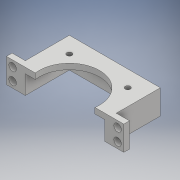
# Autodesk Inventor part: Step motor mount Top
Saved by Autodesk Inventor 2018 (Build 220112000, 112)
## iProperties
Created: 2019-03-21
Part Number: Step motor mount Top
Material: Типовые
Document SubType Name: Modeling
Designer: cosko
Density: 1 g/cm^3
Appearance: По умолчанию
Author: cosko
Autodesk Inventor part; units mm, degrees
ref_plane "YZ Plane" through (0, 0, 0) normal (1, 0, 0) x (0, 1, 0)
ref_plane "XZ Plane" through (0, 0, 0) normal (0, 1, 0) x (-1, 0, 0)
ref_plane "XY Plane" through (0, 0, 0) normal (0, 0, 1) x (1, 0, 0)
sketch "Эскиз1" plane through (0, 0, 0) normal (0, 0, 1) x (1, 0, 0)
  line L0 (-21.15, -21.15) -> (21.15, -21.15)
  line L1 (21.15, -21.15) -> (21.15, 21.15)
  line L2 (21.15, 21.15) -> (-21.15, 21.15)
  line L3 (-21.15, 21.15) -> (-21.15, -21.15)
  line L4 (-21.15, -21.15) -> (21.15, 21.15) construction
  line L5 (21.15, -21.15) -> (-21.15, 21.15) construction
  line L6 (0, 21.15) -> (15.5, 21.15) construction
  line L7 (15.5, 21.15) -> (-15.5, 21.15) construction
  line L8 (21.15, 0) -> (21.15, -15.5) construction
  line L9 (21.15, -15.5) -> (21.15, 15.5) construction
  line L10 (15.5, 21.15) -> (15.5, -21.15) construction
  line L11 (21.15, -15.5) -> (-21.15, -15.5) construction
  line L12 (21.15, 15.5) -> (-21.15, 15.5) construction
  line L13 (-15.5, 21.15) -> (-15.5, -21.15) construction
  circle A0 centre (-15.5, 15.5) radius 1.35
  circle A1 centre (-15.5, -15.5) radius 1.35
  circle A2 centre (15.5, -15.5) radius 1.35
  circle A3 centre (15.5, 15.5) radius 1.35
  circle A4 centre (0, 0) radius 11
  circle A5 centre (0, 0) radius 2.5
  circle A6 centre (0, 0) radius 2.25
  dimension "d0" = 42.3
  dimension "d1" = 42.3
  dimension "d3" = 31
  dimension "d4" = 15.5
  dimension "d5" = 31
  dimension "d6" = 2.7
  dimension "d7" = 2.7
  dimension "d8" = 2.7
  dimension "d9" = 2.7
  dimension "d10" = 22
  dimension "d11" = 5
  dimension "d12" = 4.5
  constraints: 28 end point, 16 point on line, 7 centre point, 5 perpendicular, 4 midpoint, 3 coincident, 2 parallel, 1 horizontal
  measures "d0" distance of L2.end L1.end
  measures "d1" distance of L1.end L0.end
  measures "d3" distance of L6.end L7.end
  measures "d4" distance of L8.start L8.end
  measures "d5" distance of L8.end L9.end
  measures "d6" diameter of A0
  measures "d7" diameter of A1
  measures "d8" diameter of A2
  measures "d9" diameter of A3
  measures "d10" diameter of A4
  measures "d11" diameter of A5
  measures "d12" diameter of A6
extrude "Выдавливание1" add sketch "Эскиз1" along normal blind 5 contours L3 L2 L1 L0 | A4 | A5 | A6
extrude "Выдавливание2" add sketch "Эскиз1" along normal blind 7 contours A4
extrude "Выдавливание3" add sketch "Эскиз1" along normal blind 8 contours A5
extrude "Выдавливание4" add sketch "Эскиз1" along normal blind 27 contours A6
sketch "Эскиз2" plane through (0, 0, 27) normal (0, 0, 1) x (1, 0, 0)
  line L0 (0, -1.65) -> (1.5297, -1.65)
  line L1 (0, -1.65) -> (-1.5297, -1.65)
  circle A0 centre (0, 0) radius 2.25 projected
  constraints: 4 end point, 1 point on circle, 1 point on line
extrude "Выдавливание5" cut sketch "Эскиз2" against normal blind 20 contours L0 A0 L1 picked at (0.8684, -1.7588)
sketch "Эскиз3" plane through (21.15, -21.15, 0) normal (1, 0, 0) x (0, 0, -1)
  line L0 (-8, 23.4) -> (-27, 23.4) projected
  line L1 (-8, 23.4) -> (0, 23.4) construction
  line L2 (0, 23.4) -> (0, 19.5) construction
  line L3 (0, 0) -> (0, 42.3) construction
  line L4 (-8, 19.5) -> (0, 19.5) construction
  line L5 (-8, 19.5) -> (-8, 18.9) construction
  line L6 (-8, 23.65) -> (-8, 18.65) construction
  line L7 (-8, 18.9) -> (-27, 18.9) construction
  line L8 (-27, 18.9) -> (-27, 9.3) construction
  line L9 (-27, 18.9) -> (0, 18.9) construction
  line L10 (0, 18.9) -> (0, 9.3) construction
  line L11 (0, 9.3) -> (-27, 9.3) construction
  line L12 (-27, 9.3) -> (-27, 18.9) construction
  line L13 (-27, 18.9) -> (0, 18.9)
  line L14 (0, 18.9) -> (0, 9.3)
  line L15 (0, 9.3) -> (-27, 9.3)
  line L16 (-27, 9.3) -> (-27, 18.9)
  point P0 (0, 21.15)
  dimension "d24" = 0.6
  dimension "d25" = 9.6
  constraints: 28 end point, 4 horizontal, 4 parallel, 3 perpendicular, 3 point on line, 1 vertical
  measures "d24" distance of L4.start L5.end
  measures "d25" distance of L7.end L8.end
surface extrude "ВыдавПврх1" sketch "Эскиз3" against normal up to surface (42.3 mm away) shown no curves L13 L14 L15 L16
surface_extend "Удлинить1"
surface_extend "Удлинить2"
sketch "Эскиз4" plane through (0, 0, 5) normal (0, 0, 1) x (1, 0, 0)
  line L0 (21.15, -2.25) -> (-21.15, -2.25) projected
  line L1 (21.15, 21.15) -> (-21.15, 21.15) projected
  circle A0 centre (-15.5, 15.5) radius 1.35 projected
  circle A1 centre (15.5, 15.5) radius 1.35 projected
  circle A2 centre (15.5, 15.5) radius 1.35 projected
  circle A3 centre (-15.5, 15.5) radius 1.35 projected
  circle A4 centre (-15.5, 15.5) radius 1.35 projected
  line L2 (-21.15, -2.25) -> (-21.15, 21.15)
  line L3 (21.15, 21.15) -> (21.15, -2.25)
  circle A5 centre (0, 0) radius 11 projected
  arc A6 (15.841, -2.25) -> (-15.841, -2.25) centre (0, 0) ccw
  dimension "d30" = 5
  constraints: 4 end point, 2 point on circle, 2 point on line, 1 centre point, 1 parallel, 1 vertical
  measures "d30" radial gap between concentric circles of A5 A6
extrude "Выдавливание6" add sketch "Эскиз4" along normal blind 3 separate body contours L0 A6 L2 L1 L3
sketch "Эскиз5" plane through (-21.15, -2.25, 5) normal (-1, 0, 0) x (0, 0, 1)
  line L0 (3, 23.4) -> (3, 0) projected
  line L1 (3, 0) -> (0, 0)
  line L2 (0, 0) -> (0, 3)
  line L3 (0, 3) -> (3, 3)
  line L4 (3, 3) -> (3, 0)
  point P0 (-5, 2.25)
  dimension "d33" = 3
  dimension "d34" = 3
  constraints: 8 end point, 2 parallel, 1 horizontal, 1 perpendicular
  measures "d33" distance of L2.end L3.end
  measures "d34" distance of L1.end L2.end
extrude "Выдавливание7" add sketch "Эскиз5" along normal blind 10 bodies 2
ref_plane "РабПлоскость1" through (0, -21.15, 0) normal (1, 0, 0) x (0, 0, -1)
mirror "Зеркальное отражение1" about plane through (0, -21.15, 0) normal (1, 0, 0) of "Выдавливание7" bodies 2
sketch "Эскиз6" plane through (0, 0, 5) normal (0, 0, -1) x (-1, 0, 0)
  circle A0 centre (-15.5, 15.5) radius 1.35 projected
  circle A1 centre (15.5, 15.5) radius 1.35 projected
  line L0 (-15.841, -2.25) -> (-31.15, -2.25) projected
  arc A2 (15.841, -2.25) -> (-15.841, -2.25) centre (0, 0) ccw projected
  line L1 (15.841, -2.25) -> (31.15, -2.25) projected
  line L2 (31.15, 0.75) -> (31.15, -2.25) projected
  line L3 (21.15, 0.75) -> (31.15, 0.75) projected
  line L4 (21.15, 21.15) -> (21.15, 0.75) projected
  line L5 (-21.15, 21.15) -> (21.15, 21.15) projected
  line L6 (-21.15, 0.75) -> (-21.15, 21.15) projected
  line L7 (-21.15, 0.75) -> (-31.15, 0.75) projected
  line L8 (-31.15, 0.75) -> (-31.15, -2.25) projected
  line L9 (-21.15, -21.15) -> (-21.15, 21.15) projected
  line L10 (21.15, 21.15) -> (21.15, -21.15) projected
  line L11 (-15.841, -2.25) -> (-31.15, -2.25) projected
  line L12 (-31.15, 0.75) -> (-23.4955, 0.75)
  line L13 (-23.4955, 0.75) -> (-23.4955, -2.25)
  line L14 (-23.4955, -2.25) -> (-31.15, -2.25)
  line L15 (-31.15, -2.25) -> (-31.15, 0.75)
  line L16 (15.841, -2.25) -> (31.15, -2.25) projected
  line L17 (21.15, 0.75) -> (31.15, 0.75)
  line L18 (31.15, 0.75) -> (31.15, -2.25)
  line L19 (31.15, -2.25) -> (21.15, -2.25)
  line L20 (21.15, -2.25) -> (21.15, 0.75)
  line L21 (-21.15, 0.75) -> (-31.15, 0.75) projected
  line L22 (-31.15, 0.75) -> (-21.15, 0.75)
  line L23 (-21.15, 0.75) -> (-21.15, -2.25)
  line L24 (-21.15, -2.25) -> (-31.15, -2.25)
  line L25 (-31.15, -2.25) -> (-31.15, 0.75)
  constraints: 24 end point, 6 parallel, 3 horizontal, 3 perpendicular, 2 point on line, 1 midpoint
extrude "Выдавливание8" add sketch "Эскиз6" along normal blind 10 contours L0 L13 L7 L9 | L0 L8 L7 L13 | L10 L3 L2 L1 bodies 2
sketch "Эскиз7" plane through (-31.15, 0.75, 8) normal (0, 1, 0) x (1, 0, 0)
  line L0 (10, 3) -> (10, 0) projected
  line L1 (10, 3) -> (10, 13) projected
  line L2 (0, 13) -> (10, 13) projected
  line L3 (0, 0) -> (0, 13) projected
  line L4 (10, 0) -> (0, 0) projected
  line L5 (0, 13) -> (10, 13) construction
  line L6 (5, 13) -> (5, 0) construction
  line L7 (15.309, 0) -> (0, 0) construction
  line L8 (10, 3) -> (10, 13) construction
  line L9 (10, 6.5) -> (0, 6.5) construction
  line L10 (5, 13) -> (5, 6.5) construction
  line L11 (10, 13) -> (10, 8) construction
  line L12 (10, 9.75) -> (0, 9.75) construction
  line L13 (0, 0) -> (0, 13) construction
  line L14 (5, 6.5) -> (5, 0) construction
  line L15 (10, -19) -> (10, 8) construction
  line L16 (10, 3.25) -> (0, 3.25) construction
  circle A0 centre (3.2782, 9.75) radius 2
  circle A1 centre (3.2782, 3.25) radius 2
  point P0 (31.15, 8)
  dimension "d39" = 4
  dimension "d40" = 4
  constraints: 12 end point, 6 point on line, 3 midpoint, 3 perpendicular, 2 centre point, 1 collinear
  measures "d39" diameter of A0
  measures "d40" diameter of A1
extrude "Выдавливание9" cut sketch "Эскиз7" against normal blind 8 contours A0 | A1 bodies 2
mirror "Зеркальное отражение2" about plane through (0, -21.15, 0) normal (1, 0, 0) of "Выдавливание9" bodies 2
surface_extend "Удлинить3"
surface_extend "Удлинить4"
sketch "Эскиз8" plane through (0, 0, 5) normal (0, 0, 1) x (1, 0, 0)
  line L0 (21.15, -11.85) -> (-21.15, -11.85) projected
  line L1 (-21.15, -21.15) -> (21.15, -21.15) projected
  circle A0 centre (-15.5, -15.5) radius 1.35 projected
  circle A1 centre (15.5, -15.5) radius 1.35 projected
  circle A2 centre (15.5, -15.5) radius 1.35 projected
  line L2 (-21.15, -11.85) -> (21.15, -11.85)
  line L3 (21.15, -14.85) -> (21.15, -21.15)
  line L4 (21.15, -21.15) -> (-21.15, -21.15)
  line L5 (-21.15, -21.15) -> (-21.15, -14.85)
  line L6 (0, -21.15) -> (-5, -21.15)
  line L7 (-5, -21.15) -> (5, -21.15)
  line L8 (5, -21.15) -> (-5, -21.15)
  line L9 (-5, -21.15) -> (-5, -17.15)
  line L10 (-5, -17.15) -> (5, -17.15)
  line L11 (5, -17.15) -> (5, -21.15)
  line L12 (-15.841, -2.25) -> (-31.15, -2.25) projected
  line L13 (-21.15, -11.85) -> (-28.15, -11.85)
  line L14 (21.15, -11.85) -> (28.15, -11.85)
  line L15 (-21.15, 21.15) -> (-21.15, -21.15) projected
  line L16 (-28.15, -11.85) -> (-21.15, -11.85)
  line L17 (-21.15, -11.85) -> (-21.15, -14.85)
  line L18 (-21.15, -14.85) -> (-28.15, -14.85)
  line L19 (-28.15, -14.85) -> (-28.15, -11.85)
  line L20 (21.15, -11.85) -> (28.15, -11.85)
  line L21 (28.15, -11.85) -> (28.15, -14.85)
  line L22 (28.15, -14.85) -> (21.15, -14.85)
  line L23 (21.15, -14.85) -> (21.15, -11.85)
  point P0 (0, 0)
  dimension "d45" = 5
  dimension "d46" = 10
  dimension "d47" = 4
  dimension "d48" = 7
  dimension "d49" = 7
  dimension "d50" = 3
  constraints: 40 end point, 8 parallel, 6 horizontal, 4 perpendicular, 4 point on line, 1 midpoint
  measures "d45" distance of L6.start L6.end
  measures "d46" distance of L6.end L7.end
  measures "d47" distance of L8.end L9.end
  measures "d48" distance of L0.end L13.end
  measures "d49" distance of L2.end L14.end
  measures "d50" distance of L5.end L16.end
extrude "Выдавливание10" add sketch "Эскиз8" along normal blind 3 separate body
sketch "Эскиз9" plane through (0, 0, 5) normal (0, 0, -1) x (-1, 0, 0)
  line L0 (-28.15, -14.85) -> (-28.15, -11.85) projected
  line L1 (-28.15, -11.85) -> (28.15, -11.85) projected
  line L2 (-21.15, -14.85) -> (-28.15, -14.85) projected
  line L3 (28.15, -14.85) -> (21.15, -14.85) projected
  line L4 (28.15, -11.85) -> (28.15, -14.85) projected
  line L5 (-28.15, -11.85) -> (28.15, -11.85) projected
  line L6 (-21.15, -14.85) -> (-21.15, -11.85) projected
  line L7 (21.15, -11.85) -> (21.15, -14.85) projected
  line L8 (28.15, -11.85) -> (31.15, -11.85)
  line L9 (31.15, -11.85) -> (31.15, -14.85)
  line L10 (31.15, -14.85) -> (28.15, -14.85)
  line L11 (-28.15, -14.85) -> (-31.15, -14.85)
  line L12 (-31.15, -14.85) -> (-31.15, -11.85)
  line L13 (-31.15, -11.85) -> (-28.15, -11.85)
  line L14 (-28.15, -11.85) -> (-28.15, -14.85)
  point P0 (0, 0)
  dimension "d78" = 3
  dimension "d79" = 3
  constraints: 14 end point, 3 perpendicular, 2 horizontal, 2 parallel
  measures "d78" distance of L1.end L8.end
  measures "d79" distance of L12.end L13.end
extrude "Выдавливание12" add sketch "Эскиз9" along normal blind 10 bodies 3
sketch "Эскиз10" plane through (-28.15, -14.85, 8) normal (0, -1, 0) x (1, 0, 0)
  circle A0 centre (0.2782, -9.75) radius 2 projected
  circle A1 centre (0.2782, -3.25) radius 2 projected
  circle A2 centre (0.2782, -3.25) radius 2 projected
  circle A3 centre (56.0218, -9.75) radius 2 projected
  circle A4 centre (56.0218, -3.25) radius 2 projected
  point P0 (28.15, -8)
extrude "Выдавливание13" cut sketch "Эскиз10" against normal blind 10 bodies 3
sketch "Эскиз11" plane through (0, 0, 0) normal (0, 0, -1) x (-1, 0, 0)
  line L0 (-21.15, 21.15) -> (21.15, 21.15) construction
  line L1 (0, 21.15) -> (17, 21.15) construction
  line L2 (17, 21.15) -> (21.15, 17)
  line L3 (21.15, 21.15) -> (21.15, 0.75) construction
  line L4 (0, 21.15) -> (-17, 21.15) construction
  line L5 (-17, 21.15) -> (-21.15, 17)
  line L6 (-17, 21.15) -> (-11.131, 21.15) construction
  line L7 (21.15, -21.15) -> (-21.15, -21.15) construction
  line L8 (0, -21.15) -> (-17, -21.15) construction
  line L9 (0, -21.15) -> (17, -21.15) construction
  line L10 (21.15, -21.15) -> (-21.15, -21.15) construction
  line L11 (17, -21.15) -> (21.15, -17)
  line L12 (-17, -21.15) -> (-21.15, -17)
  line L13 (-21.15, -21.15) -> (-21.15, 21.15) construction
  line L14 (-21.15, -17) -> (-21.15, -21.15) construction
  line L15 (-21.15, -21.15) -> (-17, -21.15) construction
  line L16 (-21.15, -17) -> (-21.15, -21.15)
  line L17 (-17, -21.15) -> (-21.15, -21.15)
  line L18 (21.15, 21.15) -> (21.15, -21.15) projected
  line L19 (21.15, -17) -> (21.15, -21.15)
  line L20 (21.15, -21.15) -> (17, -21.15)
  line L21 (-21.15, 21.15) -> (21.15, 21.15) projected
  line L22 (17, 21.15) -> (21.15, 21.15)
  line L23 (21.15, 21.15) -> (21.15, 17)
  line L24 (-21.15, 17) -> (-21.15, 21.15)
  line L25 (-17, 21.15) -> (-21.15, 21.15)
  point P0 (0, 0)
  dimension "d59" = 17
  dimension "d60" = 135
  dimension "d61" = 17
  dimension "d62" = 135
  dimension "d63" = 17
  dimension "d64" = 17
  constraints: 38 end point, 8 collinear, 5 point on line, 2 midpoint, 2 perpendicular, 1 equal length, 1 horizontal
  measures "d59" distance of L1.start L1.end
  measures "d60" angle of L1 L2
  measures "d61" distance of L1.start L4.end
  measures "d62" angle of L5 L6
  measures "d63" distance of L8.start L8.end
  measures "d64" distance of L8.start L9.end
extrude "Выдавливание14" cut sketch "Эскиз11" against normal up to surface (5 mm away) bodies 1
sketch "Эскиз16" plane through (0, 0, 5) normal (0, 0, -1) x (-1, 0, 0)
  line L0 (-21.15, 0.75) -> (-21.15, 21.15) projected
  line L1 (-21.15, 21.15) -> (21.15, 21.15) projected
  line L2 (-17, 21.15) -> (-21.15, 17) projected
  line L3 (21.15, 21.15) -> (21.15, 0.75) projected
  line L4 (21.15, 17) -> (17, 21.15) projected
  line L5 (-21.15, -17) -> (-17, -21.15) projected
  line L6 (-21.15, -21.15) -> (-21.15, -14.85) projected
  line L7 (21.15, -21.15) -> (-21.15, -21.15) projected
  line L8 (17, -21.15) -> (21.15, -17) projected
  line L9 (21.15, -14.85) -> (21.15, -21.15) projected
  line L10 (21.15, -21.15) -> (-21.15, -21.15) projected
  point P0 (0, 0)
  point P1 (-5, -21.15)
  point P2 (5, -21.15)
sketch "Эскиз17" plane through (0, 0, 8) normal (0, 0, 1) x (1, 0, 0)
  line L0 (-21.15, 21.15) -> (-21.15, 0.75) projected
  line L1 (21.15, 21.15) -> (-21.15, 21.15) projected
  line L2 (21.15, 0.75) -> (21.15, 21.15) projected
  line L3 (-24.15, 0.75) -> (-24.15, 24.15)
  line L4 (-24.15, 24.15) -> (24.15, 24.15)
  line L5 (24.15, 24.15) -> (24.15, 0.75)
  line L6 (-21.15, 0.75) -> (-31.15, 0.75) projected
  line L7 (-24.15, 0.75) -> (-21.15, 0.75)
  line L8 (21.15, 0.75) -> (24.15, 0.75)
  line L9 (21.15, 0.75) -> (21.15, 21.15) projected
  line L10 (21.15, 0.75) -> (21.15, 21.15)
  line L11 (21.15, 21.15) -> (-21.15, 21.15)
  line L12 (-21.15, 21.15) -> (-21.15, 0.75)
  point P0 (0, 0)
  dimension "d77" = 3
  constraints: 16 end point, 2 collinear, 1 parallel, 1 point on line, 2 other
  measures "d77" distance between parallel lines of L1 L4
sketch "Эскиз18" plane through (0, 0, 5) normal (0, 0, 1) x (1, 0, 0)
  line L0 (-28.15, -14.85) -> (-31.15, -14.85) projected
  line L1 (-31.15, -11.85) -> (-28.15, -11.85) projected
  line L2 (-41.15, -11.85) -> (-21.15, -11.85) projected
  line L3 (-31.15, -14.85) -> (-31.15, -11.85) projected
  line L4 (31.15, -11.85) -> (31.15, -14.85) projected
  line L5 (31.15, -14.85) -> (28.15, -14.85) projected
  line L6 (28.15, -11.85) -> (31.15, -11.85) projected
  line L7 (28.15, -14.85) -> (28.15, -11.85) projected
  line L8 (-28.15, -11.85) -> (-28.15, -14.85) projected
  point P0 (0, 0)
extrude "Выдавливание18" add sketch "Эскиз18" along normal blind 3 bodies 3
sketch "Эскиз20" plane through (-31.15, -14.85, -5) normal (0, -1, 0) x (1, 0, 0)
  line L0 (0, 13) -> (0, 0) projected
  line L1 (1.2939, 10) -> (3, 10) projected
  line L2 (3, 10) -> (3, 11.7306) projected
  arc A0 (1.2939, 10) -> (3, 11.7306) centre (3.2782, 9.75) ccw projected
  circle A1 centre (3.2782, 9.75) radius 2 projected
  circle A2 centre (59.0218, 9.75) radius 2 projected
  line L3 (59.3, 10) -> (59.3, 11.7306) projected
  line L4 (61.0061, 10) -> (59.3, 10) projected
  point P0 (31.15, 5)
extrude "Выдавливание19" cut sketch "Эскиз20" against normal blind 3 bodies 3
extrude "Выдавливание20" add sketch "Эскиз17" against normal up to surface (13 mm away) bodies 2
sketch "Эскиз21" plane through (0, 0, 8) normal (0, 0, 1) x (1, 0, 0)
  line L0 (21.15, -21.15) -> (21.15, -14.85) projected
  line L1 (-21.15, -21.15) -> (21.15, -21.15) projected
  line L2 (-21.15, -21.15) -> (21.15, -21.15) projected
  line L3 (-21.15, -14.85) -> (-21.15, -21.15) projected
  line L4 (-17, -21.15) -> (17, -21.15) projected
  line L5 (-17, -24.15) -> (17, -24.15)
  line L6 (5, -24.15) -> (24.15, -24.15)
  line L7 (24.15, -24.15) -> (24.15, -14.85)
  line L8 (-5, -24.15) -> (-24.15, -24.15)
  line L9 (-24.15, -24.15) -> (-24.15, -14.85)
  line L10 (21.15, -21.15) -> (-21.15, -21.15)
  line L11 (-21.15, -21.15) -> (-21.15, -14.85)
  line L12 (21.15, -14.85) -> (21.15, -21.15)
  line L13 (24.15, -14.85) -> (21.15, -14.85)
  line L14 (41.15, -11.85) -> (21.15, -11.85) projected
  line L15 (-21.15, -14.85) -> (-24.15, -14.85)
  line L16 (-41.15, -11.85) -> (-21.15, -11.85) projected
  line L17 (24.15, -14.85) -> (24.15, -24.15)
  line L18 (24.15, -24.15) -> (-24.15, -24.15)
  line L19 (-24.15, -24.15) -> (-24.15, -14.85)
  line L20 (-21.15, -14.85) -> (-31.15, -14.85) projected
  line L21 (-24.15, -14.85) -> (-21.15, -14.85)
  line L22 (-21.15, -14.85) -> (-21.15, -21.15) projected
  line L23 (-21.15, -14.85) -> (-21.15, -21.15)
  line L24 (-21.15, -21.15) -> (21.15, -21.15)
  line L25 (21.15, -21.15) -> (21.15, -14.85)
  line L26 (21.15, -14.85) -> (24.15, -14.85)
  point P0 (0, 0)
  point P1 (5, -21.15)
  point P2 (-5, -21.15)
  dimension "d86" = 3
  dimension "d87" = 3
  dimension "d88" = 3
  constraints: 36 end point, 4 collinear, 4 parallel, 4 perpendicular, 1 horizontal, 2 other
  measures "d86" distance between parallel lines of L4 L5
  measures "d87" distance between parallel lines of L1 L6
  measures "d88" distance between parallel lines of L2 L8
extrude "Выдавливание21" add sketch "Эскиз21" against normal up to surface (13 mm away) bodies 3
body "SRF1"
